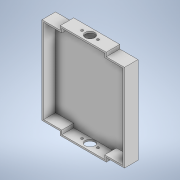
# Autodesk Inventor part: corpo2
Saved by Autodesk Inventor 2022.1 (Build 261234000, 234)
## iProperties
Created: 2021-08-03
Part Number: corpo2
Material: Generic
Document SubType Name: Modeling
Designer: nakai
Density: 1 g/cm^3
Appearance: Default
Author: nakai
Autodesk Inventor part; units mm, degrees
ref_plane "YZ Plane" through (0, 0, 0) normal (1, 0, 0) x (0, 1, 0)
ref_plane "XZ Plane" through (0, 0, 0) normal (0, 1, 0) x (-1, 0, 0)
ref_plane "XY Plane" through (0, 0, 0) normal (0, 0, 1) x (1, 0, 0)
sketch "Sketch1" plane through (0, 0, 0) normal (0, 0, 1) x (1, 0, 0)
  line L0 (0, 0) -> (58, 0)
  line L1 (58, 0) -> (58, 120)
  line L2 (58, 120) -> (0, 120)
  line L3 (0, 120) -> (0, 0)
  line L4 (58, 115) -> (81, 115)
  line L5 (81, 115) -> (81, 5)
  line L6 (81, 5) -> (58, 5)
  line L7 (58, 5) -> (58, 115)
  line L8 (0, 115) -> (-23, 115)
  line L9 (-23, 115) -> (-23, 5)
  line L10 (-23, 5) -> (0, 5)
  line L11 (0, 5) -> (0, 115)
  point P0 (0, 5)
  dimension "d0" = 58
  dimension "d1" = 120
  dimension "d20" = 23
  dimension "d21" = 5
  dimension "d22" = 5
  dimension "d26" = 23
  dimension "d27" = 5
  dimension "d28" = 5
  constraints: 24 end point, 6 parallel, 3 horizontal, 3 perpendicular, 2 point on line
  measures "d0" distance of L2.end L1.end
  measures "d1" distance of L0.end L1.end
  measures "d20" distance between parallel lines of L1 L5
  measures "d21" distance between parallel lines of L2 L4
  measures "d22" distance between parallel lines of L0 L6
  measures "d26" distance of L10.end L9.end
  measures "d27" distance between parallel lines of L2 L8
  measures "d28" distance between parallel lines of L0 L10
extrude "Extrusion1" add sketch "Sketch1" along normal blind 2
sketch "Sketch2" plane through (0, 0, 2) normal (0, 0, 1) x (1, 0, 0)
  line L0 (58, 120) -> (0, 120) projected
  line L1 (58, 0) -> (58, 120) projected
  line L2 (0, 120) -> (58, 120)
  line L3 (58, 120) -> (58, 0)
  line L4 (58, 0) -> (0, 0)
  line L5 (0, 0) -> (0, 120)
  line L6 (2, 118) -> (56, 118)
  line L7 (56, 118) -> (56, 2)
  line L8 (56, 2) -> (2, 2)
  line L9 (2, 2) -> (2, 118)
  line L10 (-23, 115) -> (-23, 5) projected
  line L11 (-23, 115) -> (2, 115)
  line L12 (2, 115) -> (2, 55.5525)
  line L13 (-23, 5) -> (-23, 115)
  line L14 (-21, 113) -> (2, 113)
  line L15 (0, 113) -> (0, 57.5525)
  line L16 (-21, 7) -> (-21, 113)
  line L17 (-21, 7) -> (2, 7)
  line L18 (-23, 5) -> (0, 5) projected
  line L19 (-23, 5) -> (2, 5)
  line L20 (81, 115) -> (58, 115) projected
  line L21 (58, 115) -> (81, 115)
  line L22 (81, 115) -> (81, 5)
  line L23 (58, 5) -> (81, 5) projected
  line L24 (81, 5) -> (58, 5)
  line L25 (56, 7) -> (79, 7)
  line L26 (79, 7) -> (79, 113)
  line L27 (79, 113) -> (56, 113)
  point P0 (0, 0)
  point P1 (0, 115)
  point P2 (2, 113)
  point P3 (2, 7)
  dimension "d4" = 2
  dimension "d5" = 2
  dimension "d6" = 2
  dimension "d7" = 2
  dimension "d30" = 2
  dimension "d31" = 2
  dimension "d32" = 2
  dimension "d33" = 2
  dimension "d34" = 2
  dimension "d35" = 2
  constraints: 44 end point, 8 perpendicular, 8 point on line, 7 parallel, 4 horizontal, 3 collinear
  measures "d4" distance between parallel lines of L0 L6
  measures "d5" distance between parallel lines of L1 L7
  measures "d6" distance between parallel lines of L4 L8
  measures "d7" distance between parallel lines of L9 L5
  measures "d30" distance between parallel lines of L10 L16
  measures "d31" distance between parallel lines of L14 L11
  measures "d32" distance between parallel lines of L17 L19
  measures "d33" distance between parallel lines of L20 L27
  measures "d34" distance between parallel lines of L22 L26
  measures "d35" distance between parallel lines of L23 L25
extrude "Extrusion2" add sketch "Sketch2" along normal blind 15 contours L1 L27 L7 L6 L9 L11 L5 L0 | L20 L22 L23 L1 L25 L26 L27 | L11 L9 L14 L5 | L5 L14 L16 L17 L18 L10 L11 | L1 L4 L5 L19 L9 L8 L7 L25 | L17 L9 L19 L5
sketch "Sketch6" plane through (0, 120, 0) normal (0, 1, 0) x (1, 0, 0)
  circle A0 centre (29, -8.5) radius 6
  circle A1 centre (39, -8.5) radius 1.5
  circle A2 centre (19, -8.5) radius 1.5
  line L0 (58, 0) -> (0, 0) projected
  line L1 (58, 0) -> (58, -17) projected
  line L2 (0, 0) -> (0, -17) projected
  dimension "d46" = 12
  dimension "d47" = 3
  dimension "d48" = 3
  dimension "d49" = 10
  dimension "d50" = 10
  dimension "d51" = 8.5
  dimension "d52" = 8.5
  dimension "d53" = 8.5
  dimension "d54" = 58
  dimension "d55" = 29
  constraints: 3 centre point
  measures "d46" diameter of A0
  measures "d47" diameter of A1
  measures "d48" diameter of A2
  measures "d49" distance of A1.centre A0.centre
  measures "d50" distance of A2.centre A0.centre
  measures "d51" distance from line of A0.centre L0
  measures "d52" distance from line of L0 A2.centre
  measures "d53" distance from line of L0 A1.centre
  measures "d54" distance between parallel lines of L1 L2
  measures "d55" distance from line of L1 A0.centre
extrude "Extrusion4" cut sketch "Sketch6" against normal up to surface (120 mm away)
equation "\"d52\" = d51"
equation "\"d53\" = d51"
equation "\"d55\" = 0.5 * d54"
body "Solid1"
